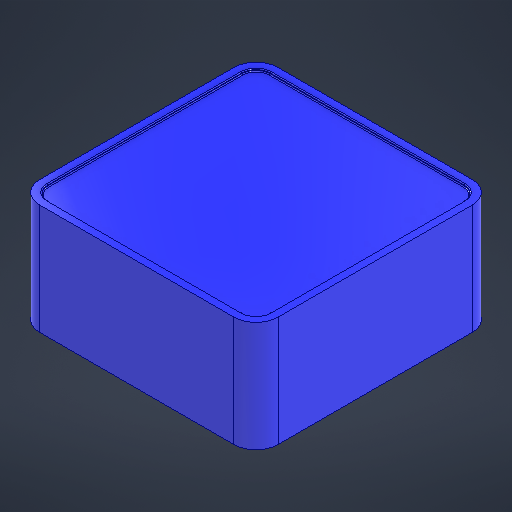
# Autodesk Inventor part: core_dummy_1
Saved by Autodesk Inventor 2026 (Build 300175000, 175)
## iProperties
Created: 2025-05-07
Part Number: core_dummy_1
Material: Generic
Document SubType Name: Modeling
Designer: Paul Juschitz
Density: 1 g/cm^3
Appearance: Blue - Wall Paint - Glossy
core_outer_width: 54,000 mm
core_outer_radius: 5,000 mm
core_height: 25,000 mm
core_inner_width: 50,400 mm
d0: 100,000 mm
d1: 100,000 mm
d5: 0,00 deg
d6: 1,800 mm
d7: 0,500 mm
d8: 0,00 deg
d9: 0,200 mm
Author: Paul Juschitz
Autodesk Inventor part; units mm, degrees
ref_plane "YZ Plane" through (0, 0, 0) normal (1, 0, 0) x (0, 1, 0)
ref_plane "XZ Plane" through (0, 0, 0) normal (0, 1, 0) x (-1, 0, 0)
ref_plane "XY Plane" through (0, 0, 0) normal (0, 0, 1) x (1, 0, 0)
sketch "Sketch1" plane through (0, 0, 0) normal (0, 1, 0) x (-1, 0, 0)
  line L0 (50, 0) -> (-50, 0)
  line L1 (0, 50) -> (0, -50)
  line L2 (22, 27) -> (-22, 27)
  arc A0 (-22, 27) -> (-27, 22) centre (-22, 22) ccw
  line L3 (-27, 22) -> (-27, -22)
  arc A1 (-27, -22) -> (-22, -27) centre (-22, -22) ccw
  line L4 (-22, -27) -> (22, -27)
  arc A2 (22, -27) -> (27, -22) centre (22, -22) ccw
  line L5 (27, -22) -> (27, 22)
  arc A3 (27, 22) -> (22, 27) centre (22, 22) ccw
  point P0 (0, 0)
  dimension "d0" = 100
  dimension "d1" = 100
  dimension "core_outer_width" = 54
  dimension "core_outer_radius" = 5
  constraints: 12 end point, 8 point on circle, 7 tangent, 4 centre point, 3 equal radius, 3 perpendicular, 2 equal length, 2 horizontal, 2 midpoint, 1 vertical, 2 other
  measures "d0" distance of L0.start L0.end
  measures "d1" distance of L1.start L1.end
  measures "core_outer_width" distance between parallel lines of L4 L2
  measures "core_outer_radius" radius of A3
extrude "Extrusion1" add sketch "Sketch1" against normal blind 25
sketch "Sketch2" plane through (0, 0, 0) normal (0, 1, 0) x (1, 0, 0)
  line L0 (-27, 22) -> (-27, -22) construction
  arc A0 (-27, -22) -> (-22, -27) centre (-22, -22) ccw construction
  line L1 (-22, -27) -> (22, -27) construction
  arc A1 (22, -27) -> (27, -22) centre (22, -22) ccw construction
  line L2 (27, -22) -> (27, 22) construction
  arc A2 (27, 22) -> (22, 27) centre (22, 22) ccw construction
  line L3 (22, 27) -> (-22, 27) construction
  arc A3 (-22, 27) -> (-27, 22) centre (-22, 22) ccw construction
  line L4 (22, -25.2) -> (-22, -25.2)
  arc A4 (-25.2, -22) -> (-22, -25.2) centre (-22, -22) ccw
  line L5 (-25.2, -22) -> (-25.2, 22)
  arc A5 (-22, 25.2) -> (-25.2, 22) centre (-22, 22) ccw
  line L6 (-22, 25.2) -> (22, 25.2)
  arc A6 (25.2, 22) -> (22, 25.2) centre (22, 22) ccw
  line L7 (25.2, 22) -> (25.2, -22)
  arc A7 (22, -25.2) -> (25.2, -22) centre (22, -22) ccw
  point P0 (0, 0)
  dimension "d6" = 1.8
  constraints: 8 end point, 8 point on circle, 4 centre point, 7 other
  measures "d6" distance between parallel lines of L1 L4
extrude "Extrusion2" cut sketch "Sketch2" against normal blind 0.5
fillet "Fillet1" radius 0.2 16 edges at (-24.2627, -0.5, -24.2627) (0, -0.5, -25.2) (24.2627, -0.5, -24.2627) (25.2, -0.5, 0) (24.2627, -0.5, 24.2627) (0, -0.5, 25.2) (-24.2627, -0.5, 24.2627) (-25.2, -0.5, 0) (-24.2627, 0, -24.2627) (0, 0, -25.2) (24.2627, 0, -24.2627) (25.2, 0, 0) (24.2627, 0, 24.2627) (0, 0, 25.2) (-24.2627, 0, 24.2627) (-25.2, 0, 0)
equation "\"d6\" = -0.5 * core_inner_width + 0.5 * core_outer_width"
equation "\"core_inner_width\" = 50.4"
body "Solid1"
